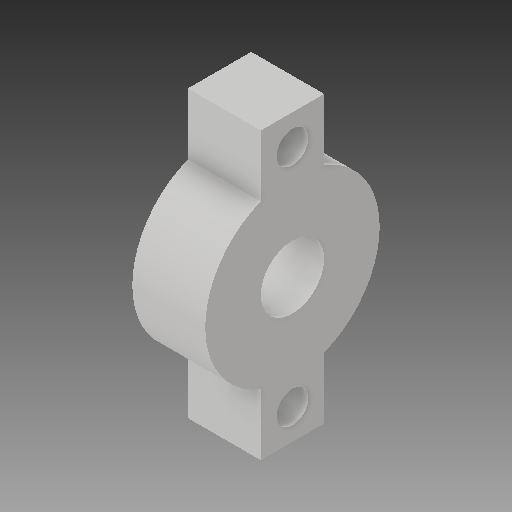
# Autodesk Inventor part: KFL004
Saved by Autodesk Inventor 2019.4 (Build 234330000, 330)
## iProperties
Created: 2019-12-11
Part Number: KFL004
Material: Generic
Document SubType Name: Modeling
Designer: Mark
Density: 1 g/cm^3
Appearance: Default
Mass: 60.4748 g
Surface Area: 138.847 cm^2
Volume: 60.4748 cm^3
Author: Mark
Autodesk Inventor part; units mm, degrees
note: some values were not read from the file. Chosen so that the rebuilt part matches the saved one: sketch regions of "Extrusion1".
ref_plane "YZ Plane" through (0, 0, 0) normal (1, 0, 0) x (0, 1, 0)
ref_plane "XZ Plane" through (0, 0, 0) normal (0, 1, 0) x (-1, 0, 0)
ref_plane "XY Plane" through (0, 0, 0) normal (0, 0, 1) x (1, 0, 0)
sketch "Sketch1" plane through (0, 0, 0) normal (1, 0, 0) x (0, 1, 0)
  circle A0 centre (0, 0) radius 10
  circle A1 centre (0, 0) radius 27.5
  circle A2 centre (35.5, 0) radius 5
  circle A3 centre (-35.5, 0) radius 5
  line L0 (-35.5, 0) -> (35.5, 0) construction
  line L1 (0, 0) -> (10, 0) construction
  line L2 (0, 0) -> (10, 0) construction
  line L3 (-45, 10) -> (45, 10)
  line L4 (45, 10) -> (45, -10)
  line L5 (45, -10) -> (-45, -10)
  line L6 (-45, -10) -> (-45, 10)
  line L7 (-45, 10) -> (45, -10) construction
  line L8 (45, 10) -> (-45, -10) construction
  dimension "d0" = 20
  dimension "d1" = 55
  dimension "d2" = 10
  dimension "d3" = 10
  dimension "d4" = 71
  dimension "d5" = 10
  dimension "d6" = 0
  dimension "d7" = 35.5
  dimension "d8" = 90
  dimension "d9" = 20
  constraints: 18 end point, 4 centre point, 4 horizontal, 2 coincident, 2 collinear, 2 midpoint, 2 parallel, 1 perpendicular
  measures "d0" diameter of A0
  measures "d1" diameter of A1
  measures "d2" diameter of A2
  measures "d3" diameter of A3
  measures "d4" distance of L0.start L0.end
  measures "d5" distance of L1.start L1.end
  measures "d6" distance between parallel lines of L1 L2
  measures "d7" distance of point (0, 0) L0.end
  measures "d8" distance of L4.end L5.end
  measures "d9" distance of L3.end L4.end
extrude "Extrusion1" add sketch "Sketch1" along normal blind 23 contours A0 L3 A1 L5 | A0 L5 A1 L3 | L3 A1 | L5 A1 | A1 L5 L6 L3 | L3 L4 L5 A1
body "Solid1"
